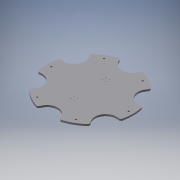
# Autodesk Inventor part: крепление2
Saved by Autodesk Inventor 2019 (Build 230136000, 136)
## iProperties
Created: 2019-10-05
Part Number: крепление2
Material: Типовые
Document SubType Name: Modeling
Designer: Iliga
Density: 1 g/cm^3
Appearance: По умолчанию
Author: Iliga
Autodesk Inventor part; units mm, degrees
ref_plane "YZ Plane" through (0, 0, 0) normal (1, 0, 0) x (0, 1, 0)
ref_plane "XZ Plane" through (0, 0, 0) normal (0, 1, 0) x (-1, 0, 0)
ref_plane "XY Plane" through (0, 0, 0) normal (0, 0, 1) x (1, 0, 0)
sketch "Эскиз7" plane through (0, 0, 0) normal (0, 1, 0) x (-1, 0, 0)
  circle A0 centre (0, 0) radius 100
  dimension "d78" = 200
  constraints: 1 centre point, 1 coincident
  measures "d78" diameter of A0
extrude "Выдавливание8" add sketch "Эскиз7" against normal blind 4
sketch "Эскиз8" plane through (0, 0, 0) normal (0, 1, 0) x (1, 0, 0)
  circle A0 centre (0, 0) radius 100 projected
  point P0 (-90, 0)
  point P1 (-45, 77.9423)
  point P2 (45, 77.9423)
  point P3 (90, 0)
  point P4 (45, -77.9423)
  point P5 (-45, -77.9423)
  dimension "d81" = 90
  dimension "d84" = 360
  constraints: 1 horizontal alignment, 7 other
  measures "d81" distance of point (0, 0) point (-90, 0)
hole "Отверстие2" at (-90, 0, 0) at (-45, 0, -77.9423) at (45, 0, -77.9423) at (90, 0, 0) at (45, 0, 77.9423) at (-45, 0, 77.9423) direction (0, -1, 0) diameter 4 depth 10
sketch "Эскиз9" plane through (0, 0, 0) normal (0, 1, 0) x (-1, 0, 0)
  point P0 (0, 0)
  point P1 (4, -38)
  point P2 (-4, -38)
  point P3 (-4, -30)
  point P4 (4, -30)
  point P5 (4, 30)
  point P6 (-4, 30)
  point P7 (-4, 38)
  point P8 (4, 38)
  dimension "d93" = 30
  dimension "d94" = 30
  dimension "d95" = 8
  dimension "d96" = 8
  dimension "d97" = 8
  dimension "d98" = 4
  constraints: 11 vertical alignment, 4 horizontal alignment
  measures "d93" vertical distance of point (0, 0) point (-4, -30)
  measures "d94" vertical distance of point (0, 0) point (-4, 30)
  measures "d95" distance of point (-4, -30) point (-4, -38)
  measures "d96" distance of point (4, -38) point (-4, -38)
  measures "d97" distance of point (-4, 30) point (-4, 38)
  measures "d98" horizontal distance of point (0, 0) point (-4, -30)
hole "Отверстие3" at (-4, 0, -38) at (4, 0, -38) at (4, 0, -30) at (-4, 0, -30) at (-4, 0, 30) at (4, 0, 30) at (4, 0, 38) at (-4, 0, 38) direction (0, -1, 0) diameter 2 depth 10
sketch "Эскиз10" plane through (0, 0, 0) normal (0, 1, 0) x (1, 0, 0)
  circle A0 centre (0, 0) radius 100 projected
  arc A1 (24.8039, -96.875) -> (-24.8039, -96.875) centre (0, -100) ccw
  dimension "d106" = 25
  dimension "d1" = 4
  dimension "d2" = 100
  dimension "d3" = 4
  dimension "d4" = 4
  dimension "d5" = 100
  dimension "d6" = 4
  dimension "d7" = 4
  dimension "d8" = 100
  dimension "d9" = 95
  dimension "d10" = 95
  dimension "d11" = 4
  dimension "d12" = 4
  dimension "d13" = 4
  dimension "d14" = 9
  dimension "d15" = 9
  dimension "d63" = 300
  dimension "d27" = 2
  dimension "d28" = 2
  dimension "d32" = 8
  dimension "d35" = 8
  dimension "d38" = 2
  dimension "d40" = 2
  dimension "d43" = 8
  dimension "d46" = 8
  dimension "d76" = 60.5
  dimension "d77" = 60.5
  constraints: 5 point on circle, 1 centre point, 1 vertical alignment
  measures "d106" radius of A1
extrude "Выдавливание9" cut sketch "Эскиз10" against normal up to next contours A1 A0 picked at (-8.0283, -92.354)
pattern_circular "Круговой массив1" count 6 over 360 about axis through (0, 0, 0) along (0, -1, 0) of "Выдавливание9"
fillet "Сопряжение1" radius 5 12 edges at (-24.8039, -2, -96.875) (24.8039, -2, -96.875) (71.4943, -2, -69.9183) (96.2982, -2, -26.9567) (71.4943, -2, 69.9183) (96.2982, -2, 26.9567) (-24.8039, -2, 96.875) (24.8039, -2, 96.875) (-71.4943, -2, 69.9183) (-96.2982, -2, 26.9567) (-96.2982, -2, -26.9567) (-71.4943, -2, -69.9183)
sketch "Эскиз6" plane through (0, 4, 0) normal (0, 1, 0) x (1, 0, 0)
  circle A0 centre (0, 0) radius 150 projected
  point P0 (90, 0)
  point P1 (45, 77.9423)
  point P2 (-45, 77.9423)
  point P3 (-90, 0)
  point P4 (-45, -77.9423)
  point P5 (45, -77.9423)
  dimension "d64" = 90
  dimension "d67" = 360
  constraints: 1 horizontal alignment, 7 other
  measures "d64" distance of A0.centre point (90, 0)
